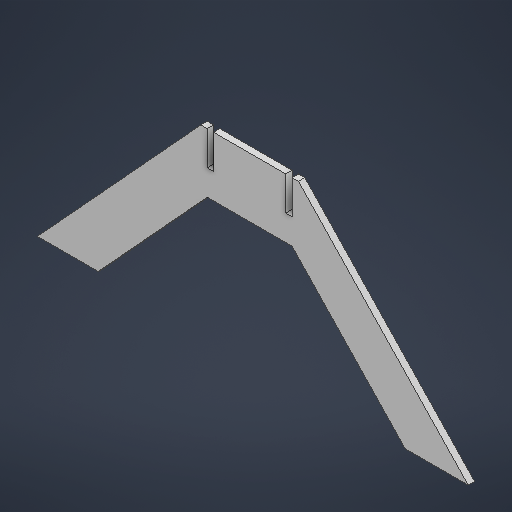
# Autodesk Inventor part: Base
Saved by Autodesk Inventor 2027 (Build 310192000, 192)
## iProperties
Created: 2026-05-24
Part Number: Base
Material: Generic
Document SubType Name: Modeling
Designer: alexy
Density: 1 g/cm^3
Appearance: Default
Author: alexy
Autodesk Inventor part; units mm, degrees
ref_plane "YZ Plane" through (0, 0, 0) normal (1, 0, 0) x (0, 1, 0)
ref_plane "XZ Plane" through (0, 0, 0) normal (0, 1, 0) x (-1, 0, 0)
ref_plane "XY Plane" through (0, 0, 0) normal (0, 0, 1) x (1, 0, 0)
sketch "Sketch1" plane through (0, 0, 0) normal (0, 0, 1) x (1, 0, 0)
  line L0 (0, 0) -> (0, 16)
  line L1 (0, 16) -> (0, 16)
  line L2 (0, 16) -> (0, 0)
  line L3 (0, 0) -> (3, 0)
  line L4 (3, 0) -> (3, 16)
  line L5 (3, 16) -> (6, 16)
  line L6 (6, 16) -> (86, -68)
  line L7 (86, -68) -> (-117, -68)
  line L8 (0, 16) -> (-34, 16)
  line L9 (-34, 16) -> (-34, 0)
  line L10 (-34, 0) -> (-37, 0)
  line L11 (-37, 0) -> (-37, 16)
  line L12 (-88.3333, -68) -> (-37, -12)
  line L13 (-37, -12) -> (3, -12)
  line L14 (3, -12) -> (56.3333, -68)
  line L15 (-37, 16) -> (-40, 16)
  line L16 (-40, 16) -> (-117, -68)
  point P0 (1.5, 0)
  dimension "d0" = 3
  dimension "d1" = 16
  dimension "d2" = 3
  dimension "d3" = 34
  dimension "d8" = 3
  dimension "d9" = 80
  dimension "d10" = 80
  dimension "d12" = 12
  dimension "d13" = 3
  dimension "d14" = 56
  constraints: 34 end point, 6 perpendicular, 4 point on line, 3 horizontal, 3 parallel, 3 vertical alignment, 2 horizontal alignment, 2 vertical, 1 coincident, 1 midpoint
  measures "d0" distance of L2.end L3.end
  measures "d1" distance of L3.end L4.end
  measures "d2" distance of L4.end L5.end
  measures "d3" distance of L1.end L8.end
  measures "d8" distance of L9.end L10.end
  measures "d9" horizontal distance of L7.end L11.end
  measures "d10" horizontal distance of L6.end L5.end
  measures "d12" distance between parallel lines of L13 L10
  measures "d13" distance of L11.end L15.end
  measures "d14" distance between parallel lines of L7 L13
extrude "Extrusion1" add sketch "Sketch1" along normal blind 3 contours L3 L4 L5 L6 L7 L14 L13 L12 L16 L15 L11 L10 L9 L8 L0
body "Solid1"
